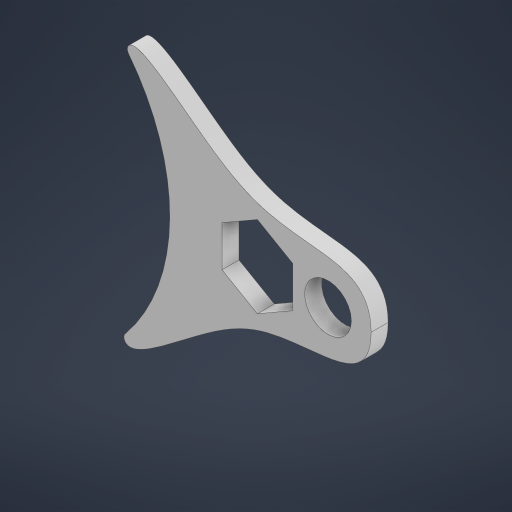
# Autodesk Inventor part: gear-interface
Saved by Autodesk Inventor 2023.2 (Build 272271000, 271)
## iProperties
Created: 2023-03-20
Part Number: gear-interface
Material: Generic
Document SubType Name: Modeling
Designer: Liam
Density: 1 g/cm^3
Appearance: Default
Author: Liam
Autodesk Inventor part; units mm, degrees
ref_plane "YZ Plane" through (0, 0, 0) normal (1, 0, 0) x (0, 1, 0)
ref_plane "XZ Plane" through (0, 0, 0) normal (0, 1, 0) x (-1, 0, 0)
ref_plane "XY Plane" through (0, 0, 0) normal (0, 0, 1) x (1, 0, 0)
sketch "Sketch1" plane through (0, 0, 0) normal (0, 0, 1) x (1, 0, 0)
  line L0 (25.3998, 3.6661) -> (28.5748, 1.833)
  line L1 (28.5748, -1.8332) -> (28.5748, 1.833)
  line L2 (28.5748, -1.8332) -> (25.3998, -3.6663)
  line L3 (22.2248, -1.8332) -> (25.3998, -3.6663)
  line L4 (22.2248, -1.8332) -> (22.2248, 1.833)
  line L5 (25.3998, 3.6661) -> (22.2248, 1.833)
  arc A0 (13.9103, 11.4928) -> (13.8254, 10.7824) centre (14.226, 11.0948) ccw
  arc A1 (13.5904, -11.0771) -> (13.7656, -11.9524) centre (13.9159, -11.4671) ccw
  arc A2 (13.5904, -11.0771) -> (13.8254, 10.7824) centre (0, 0) ccw
  circle A3 centre (31.7498, -0.0001) radius 2.0955
  line L6 (31.7498, -0.0001) -> (19.0498, -0.0001)
  line L7 (13.9103, 11.4928) -> (14.9529, 12.3199) construction
  line L8 (14.9529, 12.3199) -> (21.939, 5.9941) construction
  line L9 (21.939, 5.9941) -> (26.2427, 4.1527) construction
  line L10 (26.2427, 4.1527) -> (30.9051, 4.1527) construction
  line L11 (30.9051, 4.1527) -> (35.6157, 3.494) construction
  line L12 (35.6157, 3.494) -> (35.6157, -0.0001) construction
  spline S0 degree 4 poles (13.9103, 11.4928) (14.9529, 12.3199) (21.939, 5.9941) (26.2427, 4.1527) (30.9051, 4.1527) (35.6157, 3.494) (35.6157, -0.0001) knots 1 1 1 1 1 2 3 4 4 4 4 4
  line L13 (13.7656, -11.9524) -> (14.9529, -12.3201) construction
  line L14 (14.9529, -12.3201) -> (21.939, -5.9943) construction
  line L15 (21.939, -5.9943) -> (26.2427, -4.1529) construction
  line L16 (26.2427, -4.1529) -> (30.9051, -4.1529) construction
  line L17 (30.9051, -4.1529) -> (35.6157, -3.4942) construction
  line L18 (35.6157, -3.4942) -> (35.6157, -0.0001) construction
  spline S1 degree 4 poles (13.7656, -11.9524) (14.9529, -12.3201) (21.939, -5.9943) (26.2427, -4.1529) (30.9051, -4.1529) (35.6157, -3.4942) (35.6157, -0.0001) knots 1 1 1 1 1 2 3 4 4 4 4 4
  point P0 (0, 0)
  point P1 (16.4691, 5.9941)
  point P2 (16.469, -5.9943)
  point P3 (25.3998, -0.0001)
  dimension "d31" = 3.6662
  dimension "d32" = 3.6662
  dimension "d34" = 3.6662
  dimension "d35" = 3.6662
  dimension "d36" = 3.6662
  dimension "d37" = 3.6662
  dimension "d44" = 4.191
  constraints: 14 end point, 6 point on circle, 5 equal length, 5 symmetric about line, 4 centre point, 2 horizontal, 1 equal radius, 1 perpendicular, 1 tangent, 1 vertical, 14 other
  measures "d31" distance of point (25.4, 0) L4.end
  measures "d32" distance of L0.start point (25.4, 0)
  measures "d34" distance of L0.end point (25.4, 0)
  measures "d35" distance of L1.start point (25.4, 0)
  measures "d36" distance of L2.end point (25.4, 0)
  measures "d37" distance of point (25.4, 0) L3.start
  measures "d44" diameter of A3
extrude "Extrusion6" add sketch "Sketch1" along normal blind 1.524
equation "\"d32\" = d31"
equation "\"d34\" = d31"
equation "\"d35\" = d31"
equation "\"d36\" = d31"
equation "\"d37\" = d31"
body "Solid6"
